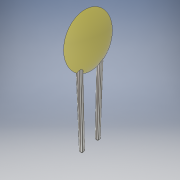
# Autodesk Inventor part: Ceramic-Capacitor
Saved by Autodesk Inventor 2018 (Build 220112000, 112)
## iProperties
Created: 2021-02-03
Part Number: Ceramic-Capacitor
Material: Všeobecné
Document SubType Name: Modeling
Designer: Jozko Mrkvicka
Density: 1 g/cm^3
Appearance: Výchozí
Author: Jozko Mrkvicka
Autodesk Inventor part; units mm, degrees
ref_plane "YZ Plane" through (0, 0, 0) normal (1, 0, 0) x (0, 1, 0)
ref_plane "XZ Plane" through (0, 0, 0) normal (0, 1, 0) x (-1, 0, 0)
ref_plane "XY Plane" through (0, 0, 0) normal (0, 0, 1) x (1, 0, 0)
sketch "Náčrt3" plane through (0, 0, 0) normal (0, 1, 0) x (-1, 0, 0)
  arc A0 (0, -2.8575) -> (0.9525, 0) centre (-3.81, 0) ccw
  arc A1 (-0.9525, 0) -> (0, -2.8575) centre (3.81, 0) ccw
  line L0 (0.9525, 0) -> (-0.9525, 0)
  point P0 (0, 0)
  constraints: 4 point on circle, 2 centre point, 2 end point
revolve "Rotace1" add sketch "Náčrt3" angle 360 about axis through (-0.9525, 0, 0) along (1, 0, 0)
sketch "Náčrt4" plane through (0, 0, 0) normal (0, 1, 0) x (-1, 0, 0)
  circle A0 centre (0, -1.27) radius 0.3175
  circle A1 centre (0, 1.27) radius 0.3175
  point P0 (0, 0)
  dimension "d6" = 0.635
  dimension "d7" = 0.635
  dimension "d8" = 2.54
  dimension "d9" = 1.27
  constraints: 2 centre point, 2 vertical alignment
  measures "d6" diameter of A0
  measures "d7" diameter of A1
  measures "d8" distance of A1.centre A0.centre
  measures "d9" distance of point (0, 0) A0.centre
extrude "Vysunutí2" add sketch "Náčrt4" along normal blind 12.7
fillet "Zaoblení1" radius 0.3175 2 edges at (0.3175, 12.7, 1.27) (0.3175, 12.7, -1.27)
